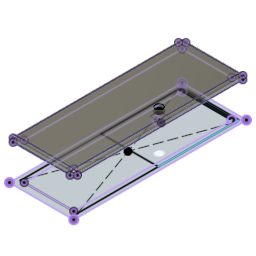
FOC-stim case v7 (Autodesk Fusion 360 design; units mm, degrees)
Autodesk Fusion 360 part; units mm, degrees
sketch "Sketch1" plane through (0, 0, 0) normal (0, 1, 0) x (1, 0, 0)
  line L0 (13.5, -43) -> (-13.5, -43)
  line L1 (-13.5, -43) -> (-13.5, 43)
  line L2 (-13.5, 43) -> (13.5, 43)
  line L3 (13.5, 43) -> (13.5, -43)
  line L4 (13.5, -43) -> (-13.5, 43) construction
  line L5 (-13.5, -43) -> (13.5, 43) construction
  line L6 (-17.5, -47) -> (-17.5, 47)
  line L7 (-17.5, 47) -> (17.5, 47)
  line L8 (17.5, 47) -> (17.5, -47)
  line L9 (17.5, -47) -> (-17.5, -47)
  dimension "d1" = 27
  dimension "d2" = 86
  dimension "d3" = -4
  constraint horizontal L0
  constraint perpendicular L0 L1
  constraint parallel L0 L2
  constraint parallel L1 L3
  constraint coincident L4 origin
  constraint coincident L5 origin
  measures "d1" distance of L1.end L2.end
  measures "d2" distance of L0.end L1.end
extrude "Extrude1" add sketch "Sketch1" along normal blind 28 makes body 1
extrude "Extrude2" add sketch "Sketch1" against normal blind 4 contours L0 L1 L2 L3 | L6 L7 L8 L9 bodies 1
ref_plane "WorkPlane1" through (0, 28, 0) normal (0, 1, 0) x (0, 0, 1)
sketch "Sketch2" plane through (0, 28, 0) normal (0, 1, 0) x (1, 0, 0)
  line L0 (15.5, 43) -> (-15.5, 43)
  line L1 (-15.5, 43) -> (-15.5, -43)
  line L2 (-15.5, -43) -> (15.5, -43)
  line L3 (15.5, -43) -> (15.5, 43)
  line L4 (15.5, 43) -> (-15.5, -43) construction
  line L5 (-15.5, 43) -> (15.5, -43) construction
  line L6 (-17.5, 47) -> (-17.5, -47)
  line L7 (-17.5, -47) -> (17.5, -47)
  line L8 (17.5, -47) -> (17.5, 47)
  line L9 (17.5, 47) -> (-17.5, 47)
  line L10 (-15.5, 43) -> (15.5, 43)
  line L11 (15.5, 43) -> (15.5, 1)
  line L12 (15.5, 1) -> (-15.5, 1)
  line L13 (-15.5, 1) -> (-15.5, 43)
  line L14 (-15.5, 43) -> (15.5, 43)
  line L15 (15.5, 43) -> (15.5, 44)
  line L16 (15.5, 44) -> (-15.5, 44)
  line L17 (-15.5, 44) -> (-15.5, 43)
  line L18 (-13.5, -43) -> (-13.5, 43)
  line L19 (13.5, 43) -> (13.5, -43)
  line L20 (13.5, -43) -> (-13.5, -43)
  line L21 (-15.5, 44) -> (15.5, 44)
  line L22 (15.5, 44) -> (15.5, 45)
  line L23 (15.5, 45) -> (-15.5, 45)
  line L24 (-15.5, 45) -> (-15.5, 44)
  point P0 (17.5, 47)
  point P1 (-17.5, 47)
  point P2 (17.5, -47)
  point P3 (-17.5, -47)
  dimension "d9" = 31
  dimension "d10" = 86
  dimension "d11" = 42
  dimension "d12" = 1
  dimension "d45" = 1
  constraint horizontal L0
  constraint perpendicular L0 L1
  constraint parallel L0 L2
  constraint parallel L1 L3
  constraint coincident L4 origin
  constraint coincident L5 origin
  constraint horizontal L10
  constraint vertical L11
  constraint horizontal L12
  constraint vertical L13
  constraint horizontal L14
  constraint vertical L15
  constraint horizontal L16
  constraint vertical L17
  constraint horizontal L21
  constraint vertical L22
  constraint horizontal L23
  constraint vertical L24
  measures "d9" distance of L1.end L2.end
  measures "d10" distance of L0.end L1.end
  measures "d11" distance of L0.end L12.end
  measures "d12" distance of L0.end L16.end
  measures "d45" distance of L16.end L23.end
extrude "Extrude3" add sketch "Sketch2" along normal blind 20 contours L0 L3 L10 L11 L12 L14 L19 | L0 L10 L14 L15 L16 L17 L21 | L2 L3 L12 L19 | L16 L21 L22 L23 L24 | L0 L1 L10 L12 L13 L14 L18 | L1 L2 L12 L18 | L6 L7 L8 L9 bodies 1
extrude "Extrude7" cut sketch "Sketch2" along normal blind 10 contours L0 L3 L10 L11 L12 L14 L19 | L0 L10 L14 L15 L16 L17 L21 | L0 L1 L10 L12 L13 L14 L18 bodies 1
chamfer "Chamfer1" distance 8 distance2 2 2 edges at (-13.5, 38, -22) (13.5, 38, -22) measured on face at (-13.5, 25.3333, 28.3333) measured on face at (13.5, 25.3333, 28.3333) on bodies 1
chamfer "Chamfer2" distance 1 angle 45 1 edges at (0, 38, -44) on bodies 1
sketch "Sketch3" plane through (0, 0, -47) normal (0, 0, -1) x (-1, 0, 0)
  line L0 (17.5, -4) -> (17.5, 48)
  line L1 (17.5, 48) -> (-17.5, 48)
  line L2 (-17.5, 48) -> (-17.5, -4)
  line L3 (-17.5, -4) -> (17.5, -4)
  line L4 (-15.5, 28) -> (-8, 28) construction
  line L5 (-8, 28) -> (-8, 31.5) construction
  line L6 (-8, 31.5) -> (-15.5, 31.5) construction
  line L7 (-15.5, 31.5) -> (-15.5, 28) construction
  line L8 (-10.5, 30) -> (-5.5, 30)
  arc A0 (-5.5, 30) -> (-5.5, 33) centre (-5.5, 31.5) ccw
  line L9 (-5.5, 33) -> (-10.5, 33)
  arc A1 (-10.5, 33) -> (-10.5, 30) centre (-10.5, 31.5) ccw
  line L10 (-10.5, 31.5) -> (-5.5, 31.5) construction
  line L11 (-15.5, 28) -> (15.5, 28)
  line L12 (15.5, 28) -> (5.5, 28) construction
  line L13 (5.5, 28) -> (5.5, 40) construction
  line L14 (5.5, 40) -> (15.5, 40) construction
  line L15 (15.5, 40) -> (15.5, 28) construction
  circle A2 centre (5.5, 40) radius 4
  arc A3 (-10.5, 36) -> (-10.5, 27) centre (-10.5, 31.5) ccw
  line L16 (-10.5, 27) -> (-5.5, 27)
  arc A4 (-5.5, 27) -> (-5.5, 36) centre (-5.5, 31.5) ccw
  line L17 (-5.5, 36) -> (-10.5, 36)
  circle A5 centre (5.5, 40) radius 5.5
  point P0 (-8, 31.5)
  dimension "d15" = 7.5
  dimension "d16" = 3.5
  dimension "d17" = 3
  dimension "d39" = 10
  dimension "d40" = 12
  dimension "d41" = 8
  dimension "d44" = 3
  dimension "d82" = 1.5
  dimension "d85" = 5
  constraint horizontal L4
  constraint vertical L5
  constraint horizontal L6
  constraint vertical L7
  constraint coincident L4.start L7.end
  constraint tangent L8 A0
  constraint tangent A0 L9
  constraint parallel L8 L9
  constraint tangent L9 A1
  constraint tangent L8 A1
  constraint perpendicular L5 L10
  constraint coincident P0 L5.end
  constraint midpoint L10 P0
  constraint horizontal L12
  constraint vertical L13
  constraint horizontal L14
  constraint vertical L15
  constraint coincident L11.end L12.start
  constraint coincident L13.end L14.start
  measures "d15" distance of L4.start L4.end
  measures "d16" distance of L4.start L6.end
  measures "d17" diameter of A0
  measures "d39" distance of L11.end L12.end
  measures "d40" distance of L11.end L14.end
  measures "d41" diameter of A2
  measures "d44" distance of A1
  measures "d85" distance of A1.centre A0.centre
extrude "Extrude4" cut sketch "Sketch3" against normal blind 5 contours L8 A0 L9 A1 bodies 1
fillet "Fillet1" radius 2 8 edges at (17.5, 22, -47) (-17.5, 22, -47) (17.5, 22, 47) (-17.5, 22, 47) (-17.5, -4, 0) (0, -4, 47) (17.5, -4, 0) (0, -4, -47) on bodies 1
sketch "Sketch4" plane through (17.5, 0, 0) normal (1, 0, 0) x (0, 0, -1)
  line L0 (-45, 48) -> (-45, -2)
  line L1 (-45, -2) -> (45, -2)
  line L2 (45, -2) -> (45, 48)
  line L3 (45, 48) -> (-45, 48)
  line L4 (-38, 5) -> (38, 5) construction
  line L5 (38, 5) -> (38, 41) construction
  line L6 (38, 41) -> (-38, 41) construction
  line L7 (-38, 41) -> (-38, 5) construction
  circle A0 centre (-38, 41) radius 2.5
  circle A1 centre (-38, 41) radius 2.7
  circle A2 centre (0, 41) radius 2.7
  circle A3 centre (0, 41) radius 2.5
  circle A4 centre (38, 41) radius 2.7
  circle A5 centre (38, 41) radius 2.5
  circle A6 centre (-38, 4) radius 2.7
  circle A7 centre (-38, 4) radius 2.5
  circle A8 centre (0, 4) radius 2.7
  circle A9 centre (0, 4) radius 2.5
  circle A10 centre (38, 4) radius 2.7
  circle A11 centre (38, 4) radius 2.5
  dimension "d22" = -7
  dimension "d23" = 5
  dimension "d24" = 0.2
  dimension "d27" = 76
  dimension "d28" = -37
  constraint coincident L6.end L7.start
  measures "d23" diameter of A0
extrude "Extrude5" add sketch "Sketch4" along normal blind 2 draft -10 contours A0 | A3 | A5 | A7 | A9 | A11 bodies 1
extrude "Extrude6" cut sketch "Sketch4" along normal blind 1.5 draft -10 from surface at -35 contours A0 | A1 | A2 | A3 | A4 | A5 | A6 | A7 | A8 | A9 | A10 | A11 bodies 1
extrude "Extrude8" cut sketch "Sketch3" against normal up to surface (4 mm away) draft -2 contours A2 bodies 1
extrude "Extrude9" cut sketch "Sketch2" along normal blind 5 contours L16 L21 L22 L23 L24 bodies 1
chamfer "Chamfer3" distance 1 angle 45 2 edges at (13, 33, -45) (-5, 33, -45) on bodies 1
extrude "Extrude10" cut sketch "Sketch3" against normal blind 1 contours L11 A3 A4 L17 | L11 A3 L16 A4 bodies 1
chamfer "Chamfer4" distance 1 distance2 2 4 edges at (1, 31.5, -46) (8, 27, -46) (15, 31.5, -46) (8, 36, -46) measured on face at (1.3982, 33.3508, -46.6667) measured on face at (8.8333, 27, -46.6667) measured on face at (10.7243, 27.0056, -46.3333) measured on face at (7.1667, 36, -46.6667) on bodies 1
sketch "Sketch5" plane through (0, 0, 47) normal (0, 0, 1) x (1, 0, 0)
  line L0 (-15.5, 48) -> (-15.5, -2)
  line L1 (-15.5, -2) -> (15.5, -2)
  line L2 (15.5, -2) -> (15.5, 48)
  line L3 (15.5, 48) -> (-15.5, 48)
  circle A0 centre (-5.5, 40) radius 3.25
  circle A1 centre (-5.5, 40) radius 4.25
  circle A2 centre (-5.5, 40) radius 7.75
  point P0 (-5.5, 40)
  dimension "d53" = 6.5
  dimension "d54" = 1
  dimension "d77" = 4.5
  constraint coincident P0 A0.centre
  measures "d53" diameter of A0
extrude "Extrude11" cut sketch "Sketch5" along normal up to surface (2.5 mm away) draft 10 from surface at -2.5 contours A0 | A1 bodies 1
extrude "Extrude12" cut sketch "Sketch5" against normal up to surface (1.5 mm away) from surface at -2.5 contours A0 bodies 1
extrude "Extrude13" cut sketch "Sketch2" along normal mid plane 6 from surface at 9.0002 contours L2 L3 L12 L19 | L1 L2 L12 L18 bodies 1
chamfer "Chamfer5" distance 5 distance2 1.5 2 edges at (14.5, 28, -1) (-14.5, 28, -1) measured on face at (14.8333, 30.0001, -1) measured on face at (-14.8333, 32.0001, -1) on bodies 1
chamfer "Chamfer6" distance 5.9 distance2 2 2 edges at (-13.5, 40, 21) (13.5, 40, 21) measured on face at (-13.5, 44.6662, 28.3333) measured on face at (13.5, 44.6662, 28.3333) on bodies 1
sketch "Sketch6" plane through (0, 48, 0) normal (0, 1, 0) x (-1, 0, 0)
  arc A0 (17.5, 45) -> (15.5, 47) centre (15.5, 45) ccw
  line L0 (15.5, 47) -> (-15.5, 47)
  arc A1 (-15.5, 47) -> (-17.5, 45) centre (-15.5, 45) ccw
  line L1 (-17.5, 45) -> (-17.5, -45)
  arc A2 (-17.5, -45) -> (-15.5, -47) centre (-15.5, -45) ccw
  line L2 (-15.5, -47) -> (15.5, -47)
  arc A3 (15.5, -47) -> (17.5, -45) centre (15.5, -45) ccw
  line L3 (17.5, -45) -> (17.5, 45)
  line L4 (-13.5, -43) -> (-13.5, 43)
  line L5 (-13.5, 43) -> (13.5, 43)
  line L6 (13.5, 43) -> (13.5, -43)
  line L7 (13.5, -43) -> (-13.5, -43)
  line L8 (-15.5, -2.5) -> (-13.5, -2.5)
  line L9 (-15.5, -2.5) -> (-9.5, -2.5) construction
  line L10 (-9.5, -2.5) -> (-9.5, -7.5) construction
  line L11 (-9.5, -7.5) -> (-15.5, -7.5) construction
  line L12 (-15.5, -7.5) -> (-15.5, -2.5) construction
  circle A4 centre (-9.5, -7.5) radius 2
  dimension "d70" = 6
  dimension "d71" = 5
  dimension "d72" = 4
  constraint horizontal L9
  constraint vertical L10
  constraint horizontal L11
  constraint vertical L12
  constraint coincident L8.start L9.start
  constraint coincident L10.end L11.start
  measures "d70" distance of L8.start L9.end
  measures "d71" distance of L8.start L11.end
  measures "d72" diameter of A4
extrude "Extrude14" add sketch "Sketch6" along normal blind 2 separate body contours A0 L0 A1 L1 A2 L2 A3 L3 | L4 L5 L6 L7 makes body 2
extrude "Extrude15" add sketch "Sketch6" against normal blind 3 draft -1 contours L4 L5 L6 L7 bodies 2
fillet "Fillet2" radius 2 8 edges at (0, 50, 47) (16.9142, 50, 46.4142) (17.5, 50, 0) (16.9142, 50, -46.4142) (0, 50, -47) (-16.9142, 50, -46.4142) (-17.5, 50, 0) (-16.9142, 50, 46.4142) on bodies 2
extrude "Extrude17" cut sketch "Sketch3" against normal blind 1 contours A5 bodies 1
extrude "Extrude18" cut sketch "Sketch5" along normal up to surface contours A0 | A1 | A2 end surface through (-13.5, 48, -43) normal (0, -0.017452, -0.999848) offset 0 bodies 2
hidden bodies 1
